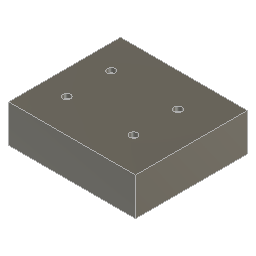
Крепление аккамулятора FengBao (Autodesk Fusion 360 design; units mm, degrees)
Autodesk Fusion 360 part; units mm, degrees
sketch "Sketch1" plane through (0, 0, 0) normal (0, 0, 1) x (1, 0, 0)
  line L0 (26, 17) -> (-26, 17)
  line L1 (-26, 17) -> (-26, -17)
  line L2 (-26, -17) -> (26, -17)
  line L3 (26, -17) -> (26, 17)
  line L4 (-26, 17) -> (26, -17) construction
  line L5 (26, 20.125) -> (-26, 20.125)
  line L6 (-26, 20.125) -> (-26, -20.125)
  line L7 (-26, -20.125) -> (26, -20.125)
  line L8 (26, -20.125) -> (26, 20.125)
  line L9 (-26, 20.125) -> (26, -20.125) construction
  line L10 (26, -20.125) -> (31, -20.125)
  line L11 (31, -20.125) -> (31, 0)
  line L12 (1.75, 0) -> (22.5, 0)
  line L13 (31, 20.125) -> (31, 0)
  line L14 (26, 20.125) -> (31, 20.125)
  line L15 (-26, -20.125) -> (-26, -25.125)
  line L16 (-26, -25.125) -> (31, -25.125)
  line L17 (31, -25.125) -> (31, -20.125)
  line L18 (-26, 25.125) -> (31, 25.125)
  line L19 (31, 25.125) -> (31, 20.125)
  line L20 (-26, 20.125) -> (-26, 25.125)
  dimension "d1" = 52
  dimension "d2" = 34
  dimension "d3" = 52
  dimension "d4" = 40.25
  dimension "d7" = 5
  constraint horizontal L0
  constraint perpendicular L0 L1
  constraint parallel L0 L2
  constraint parallel L1 L3
  constraint coincident L4 origin
  constraint horizontal L5
  constraint perpendicular L5 L6
  constraint parallel L5 L7
  constraint parallel L6 L8
  constraint coincident L9 origin
  constraint perpendicular L8 L10
  constraint perpendicular L10 L11
  constraint symmetric L7.end L12 L5.start
  constraint symmetric L10.end L12 L13.start
  constraint symmetric L11.end L12 L13.end
  constraint perpendicular L7 L15
  constraint perpendicular L15 L16
  constraint perpendicular L10 L17
  constraint symmetric L6.end L12 L5.end
  constraint symmetric L12 L15.end L18.start
  constraint symmetric L12 L16.end L18.end
  measures "d1" distance of L1.end L2.end
  measures "d2" distance of L0.end L1.end
  measures "d3" distance of L6.end L7.end
  measures "d4" distance of L5.end L6.end
  measures "d7" distance of L6.end L15.end
extrude "Extrude1" add sketch "Sketch1" along normal blind 5.2 contours L3 L8 L10 L11 L13 L14 | L0 L5 L6 L8 | L2 L6 L7 L8 | L5 L14 L18 L19 L20 | L7 L10 L15 L16 L17
extrude "Extrude2" add sketch "Sketch1" along normal blind 14 contours L3 L8 L10 L11 L13 L14 | L5 L14 L18 L19 L20 | L7 L10 L15 L16 L17
extrude "Extrude3" add sketch "Sketch1" along normal blind 17 and the other way blind -14
sketch "Sketch2" plane through (0, 0, 17) normal (0, 0, 1) x (-1, 0, 0)
  line L0 (26, -25.125) -> (26, 25.125)
  line L1 (26, 25.125) -> (-31, 25.125)
  line L2 (-31, 25.125) -> (-31, -25.125)
  line L3 (-31, -25.125) -> (26, -25.125)
  circle A0 centre (15, 10) radius 1.75
  circle A1 centre (-15, 10) radius 1.75
  line L4 (-1.75, 0) -> (-22.5, 0)
  circle A2 centre (-15, -10) radius 1.75
  circle A3 centre (15, -10) radius 1.75
  dimension "d14" = 3.5
  dimension "d15" = 3.5
  constraint symmetric A0 L4 A3
  constraint symmetric A1 L4 A2
  measures "d14" diameter of A0
  measures "d15" diameter of A1
extrude "Extrude4" cut sketch "Sketch2" against normal blind 5 contours A0 | A1 | A2 | A3
chamfer "Chamfer1" distance 1 angle 45 4 edges at (-13.3684, 10.6328, 14) (-13.3684, -9.3672, 14) (16.6316, 10.6328, 14) (16.6316, -9.3672, 14)
chamfer "Chamfer2" distance 1 angle 45 2 edges at (-26, 17, 2.6) (-26, -17, 2.6)
chamfer "Chamfer3" distance 1 angle 45 2 edges at (-26, 19.0625, 5.2) (-26, -19.0625, 5.2)
